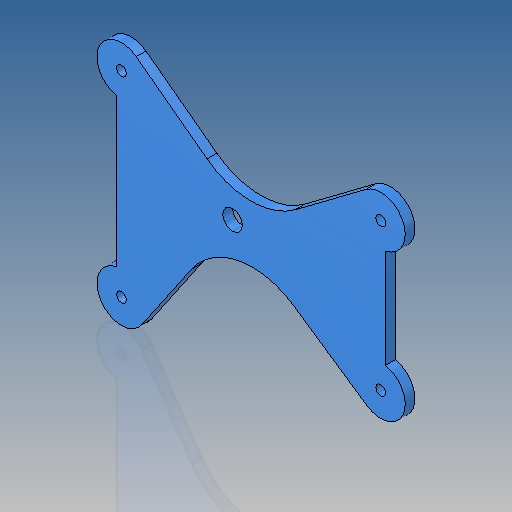
# Autodesk Inventor part: Protector
Saved by Autodesk Inventor 2017 (Build 210142000, 142)
## iProperties
Part Number: Protector
Material: Genérico
Document SubType Name: Modeling
Designer: Leo
Density: 1 g/cm^3
Appearance: Cian
Description: Aluminio compuesto routeado CNC
Author: Leo
Autodesk Inventor part; units mm, degrees
ref_plane "YZ Plane" through (0, 0, 0) normal (1, 0, 0) x (0, 1, 0)
ref_plane "XZ Plane" through (0, 0, 0) normal (0, 1, 0) x (-1, 0, 0)
ref_plane "XY Plane" through (0, 0, 0) normal (0, 0, 1) x (1, 0, 0)
sketch "Boceto1" plane through (0, 0, 0) normal (0, 0, 1) x (1, 0, 0)
  circle A0 centre (22.1541, -50) radius 2 projected
  circle A1 centre (127.9669, -30) radius 2 projected
  circle A2 centre (127.9669, 30) radius 2 projected
  line L0 (93.0368, 16.347) -> (121.9748, 38.0059)
  arc A3 (129.9669, 20.202) -> (121.9748, 38.0059) centre (127.9669, 30) ccw
  line L1 (129.9669, 20.202) -> (129.9669, -20.202)
  arc A4 (122.3322, -38.2613) -> (129.9669, -20.202) centre (127.9669, -30) ccw
  line L2 (122.3322, -38.2613) -> (92.471, -17.894)
  line L3 (50.7827, -25.7736) -> (30.4154, -55.6348)
  arc A5 (20.1541, -40.202) -> (30.4154, -55.6348) centre (22.1541, -50) ccw
  circle A6 centre (67.5, 0) radius 4 projected
  arc A7 (92.471, -17.894) -> (50.7827, -25.7736) centre (75.5667, -42.6779) ccw
  circle A8 centre (22.1541, 30) radius 2
  arc A9 (57.0842, 16.347) -> (93.0368, 16.347) centre (75.0605, 40.3647) ccw
  line L4 (57.0842, 16.347) -> (28.1462, 38.0059)
  arc A10 (28.1462, 38.0059) -> (20.1541, 20.202) centre (22.1541, 30) ccw
  line L5 (20.1541, 20.202) -> (20.1541, -40.202)
  point P0 (0, 0)
  point P1 (67.6871, -0.9897)
  dimension "d0" = 10
  dimension "d1" = 8
  dimension "d4" = 10
  dimension "d5" = 30
  dimension "d6" = 8
  dimension "d7" = 90
  constraints: 12 end point, 12 point on circle, 8 tangent, 7 centre point, 4 concentric, 4 equal radius, 3 equal length, 2 point on line, 2 vertical, 1 horizontal alignment, 1 vertical alignment
  measures "d0" radius of A3
  measures "d1" distance edge to line of A3 L1
  measures "d4" radius of A5
  measures "d5" radius of A7
  measures "d6" distance edge to line of A10 L5
  measures "d7" angle of L3 L2
extrude "Extrusión1" add sketch "Boceto1" along normal blind 4
equation "\"d4\" = d0"
equation "\"d6\" = d1"
